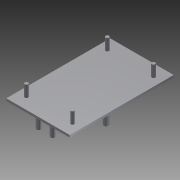
# Autodesk Inventor part: line sensor
Saved by Autodesk Inventor 2012 (Build 160160000, 160)
## iProperties
Created: 2012-11-30
Part Number: line sensor
Material: Default
Document SubType Name: Modeling
Designer: irwan
Density: 1 g/cm^3
Author: irwan
Autodesk Inventor part; units mm, degrees
ref_plane "YZ Plane" through (0, 0, 0) normal (1, 0, 0) x (0, 1, 0)
ref_plane "XZ Plane" through (0, 0, 0) normal (0, 1, 0) x (-1, 0, 0)
ref_plane "XY Plane" through (0, 0, 0) normal (0, 0, 1) x (1, 0, 0)
sketch "Sketch1" plane through (0, 0, 0) normal (0, 0, 1) x (1, 0, 0)
  line L0 (-25.9313, 51.336) -> (29.0687, 51.336)
  line L1 (29.0687, 51.336) -> (29.0687, -38.664)
  line L2 (29.0687, -38.664) -> (-25.9313, -38.664)
  line L3 (-25.9313, -38.664) -> (-25.9313, 51.336)
  circle A0 centre (-4.4697, 44.536) radius 2
  circle A1 centre (-18.7076, 12.736) radius 2
  circle A2 centre (-9.9812, 12.736) radius 2
  circle A3 centre (-4.4697, -18.464) radius 2
  line L4 (1.5687, -29.464) -> (-8.4313, -29.464)
  line L5 (-8.4313, -29.464) -> (-8.4313, -38.664)
  circle A4 centre (7.6071, 44.536) radius 2
  circle A5 centre (21.8451, 12.736) radius 2
  circle A6 centre (13.1186, 12.736) radius 2
  circle A7 centre (7.6071, -18.464) radius 2
  line L6 (1.5687, -29.464) -> (11.5687, -29.464)
  line L7 (11.5687, -29.464) -> (11.5687, -38.664)
  circle A8 centre (21.5687, 41.336) radius 1.5
  circle A9 centre (-18.4313, 41.336) radius 1.5
  circle A10 centre (21.5687, -28.664) radius 1.5
  circle A11 centre (-18.4313, -28.664) radius 1.5
  point P0 (0, 0)
  point P1 (3.1375, 0)
  dimension "d0" = 55
  dimension "d1" = 90
  dimension "d2" = 4
  dimension "d3" = 6.8
  dimension "d4" = 4
  dimension "d5" = 4
  dimension "d6" = 38.6
  dimension "d7" = 38.6
  dimension "d8" = 4
  dimension "d9" = 69.8
  dimension "d10" = 10
  dimension "d11" = 80.8
  dimension "d18" = 3
  dimension "d19" = 7.5
  dimension "d20" = 10
  dimension "d21" = 3
  dimension "d22" = 10
  dimension "d23" = 7.5
  dimension "d24" = 3
  dimension "d25" = 7.5
  dimension "d26" = 10
  dimension "d27" = 3
  dimension "d28" = 7.5
  dimension "d29" = 10
  constraints: 16 end point, 12 centre point, 3 perpendicular, 2 parallel, 2 point on line, 1 horizontal
  measures "d0" distance of L1.end L2.end
  measures "d1" distance of L0.end L1.end
  measures "d2" diameter of A0
  measures "d3" distance from line of A0.centre L0
  measures "d4" diameter of A1
  measures "d5" diameter of A2
  measures "d6" distance from line of A1.centre L0
  measures "d7" distance from line of A2.centre L0
  measures "d8" diameter of A3
  measures "d9" distance from line of A3.centre L0
  measures "d10" distance of L4.start L4.end
  measures "d11" distance between parallel lines of L4 L0
  measures "d18" diameter of A8
  measures "d19" distance from line of L1 A8.centre
  measures "d20" distance from line of L0 A8.centre
  measures "d21" diameter of A9
  measures "d22" distance from line of L0 A9.centre
  measures "d23" distance from line of L3 A9.centre
  measures "d24" diameter of A10
  measures "d25" distance from line of L1 A10.centre
  measures "d26" distance from line of L2 A10.centre
  measures "d27" diameter of A11
  measures "d28" distance from line of L3 A11.centre
  measures "d29" distance from line of L2 A11.centre
extrude "Extrusion1" add sketch "Sketch1" along normal blind 2 contours L0 L1 L2 L7 L6 L4 L5 L3 | A8 | A9 | A10 | A11
extrude "Extrusion2" add sketch "Sketch1" along normal blind 15 contours A0 | A1 | A2 | A3 | A4 | A5 | A6 | A7
extrude "Extrusion3" add sketch "Sketch1" along normal blind 7 contours L5 L4 L6 L7 L2
extrude "Extrusion4" add sketch "Sketch1" against normal blind 10 contours A8
extrude "Extrusion5" add sketch "Sketch1" against normal blind 10 contours A9
extrude "Extrusion6" add sketch "Sketch1" against normal blind 10 contours A10 | A11
body "Solid1"
